Rolling 4x13x5 (Autodesk Fusion 360 design; units mm, degrees)
Autodesk Fusion 360 part; units mm, degrees
sketch "Sketch1" plane through (0, 0, 0) normal (0, 0, 1) x (1, 0, 0)
  circle A0 centre (0, 0) radius 6.5
  circle A1 centre (0, 0) radius 2
  circle A2 centre (0, 0) radius 5.5
  circle A3 centre (0, 0) radius 3
  dimension "d1" = 13
  dimension "d2" = 4
  dimension "d5" = -1
  dimension "d6" = 1
  constraint coincident A0.centre A1.centre
  measures "d1" diameter of A0
  measures "d2" diameter of A1
extrude "Extrude2" add sketch "Sketch1" along normal blind 5 contours A0 makes body 1
fillet "Fillet1" radius 0.2 2 edges at (-6.0601, -2.3505, 5) (-5.1278, 1.9889, 5) on bodies 1
fillet "Fillet1" radius 0.2 2 edges at (-6.0601, -2.3505, 0) (-5.1278, 1.9889, 0) on bodies 1
extrude "Extrude3" add sketch "Sketch1" along normal blind 5 separate body contours A3 makes body 2
fillet "Fillet2" radius 0.2 2 edges at (-2.797, -1.0848, 5) (-1.8647, 0.7232, 5) on bodies 2
fillet "Fillet2" radius 0.2 2 edges at (-2.797, -1.0848, 0) (-1.8647, 0.7232, 0) on bodies 2
extrude "Extrude4" add sketch "Sketch1" along normal blind 5 separate body contours A2 makes body 3
fillet "Fillet3" radius 0.2 2 edges at (-5.1278, -1.9889, 5) (-2.797, 1.0848, 5) on bodies 3
fillet "Fillet3" radius 0.2 2 edges at (-5.1278, -1.9889, 0) (-2.797, 1.0848, 0) on bodies 3
combine "Combine1" operation add target body 1 tool bodies 2 3
